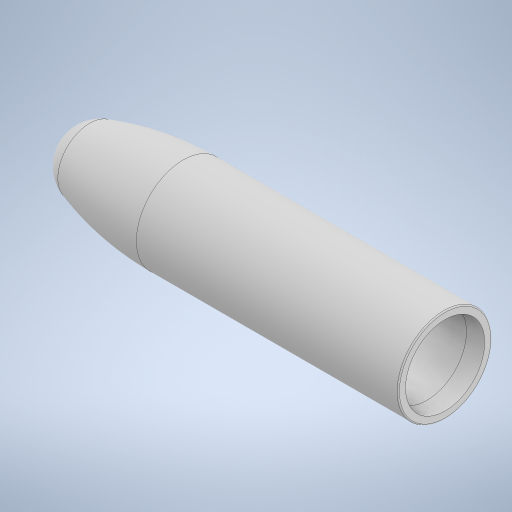
# Autodesk Inventor part: Cap
Saved by Autodesk Inventor 2024 (Build 280153000, 153)
## iProperties
Created: 2024-10-19
Part Number: Cap
Material: Generic
Document SubType Name: Modeling
Designer: Emil
Density: 1 g/cm^3
Appearance: Default
Author: Emil
Autodesk Inventor part; units mm, degrees
ref_plane "YZ Plane" through (0, 0, 0) normal (1, 0, 0) x (0, 1, 0)
ref_plane "XZ Plane" through (0, 0, 0) normal (0, 1, 0) x (-1, 0, 0)
ref_plane "XY Plane" through (0, 0, 0) normal (0, 0, 1) x (1, 0, 0)
sketch "Sketch1" plane through (0, 0, 0) normal (0, 0, 1) x (1, 0, 0)
  line L0 (-32.3906, 7.996) -> (-32.3906, -0.004) construction
  line L1 (-40.3906, -0.004) -> (-32.3906, -0.004) construction
  line L2 (61.6987, -0.004) -> (-73.3826, -0.004) construction
  line L3 (24.6094, 8.046) -> (24.6094, 6.796)
  line L4 (-40.3906, -0.004) -> (-39.1406, -0.004)
  line L5 (21.2094, 9.588) -> (21.2094, 3.996) construction
  line L6 (24.6094, 6.796) -> (21.4757, 6.7961)
  line L7 (24.6094, 8.046) -> (-20.3906, 8.046)
  line L8 (-40.3906, -0.004) -> (-40.3906, 3.996)
  arc A0 (-20.3906, 8.046) -> (-40.3906, 3.996) centre (-20.3906, -43.3617) ccw
  line L9 (20.9432, 6.7961) -> (-22.0568, 6.7961)
  line L10 (-39.1406, -0.004) -> (-39.1406, 2.996)
  arc A1 (-22.0568, 6.7961) -> (-39.1406, 2.996) centre (-20.84, -38.9748) ccw
  line L11 (20.9432, 6.7961) -> (21.4757, 6.7961)
  point P0 (0, 0)
  point P1 (-32.3906, 6.746)
  dimension "d3" = 1.25
  dimension "d4" = 65
  dimension "d6" = 6.8
  dimension "d7" = 8.05
  dimension "d8" = 3.4
  dimension "d12" = 45
  dimension "d13" = 4
  dimension "d14" = 3
  dimension "d16" = 43
  constraints: 24 end point, 5 horizontal, 4 point on circle, 4 vertical, 3 point on line, 2 centre point, 1 collinear, 1 horizontal alignment, 1 tangent
  measures "d3" distance of L3.start L3.end
  measures "d4" horizontal distance of L3.start L1.start
  measures "d6" distance from line of L2 L3.end
  measures "d7" distance from line of L2 L3.start
  measures "d8" distance between parallel lines of L3 L5
  measures "d12" distance of L3.start L7.end
  measures "d13" distance of L1.start L8.end
  measures "d14" distance of L4.end L10.end
  measures "d16" distance of L9.start L9.end
revolve "Revolution1" add sketch "Sketch1" angle 360 about axis through (61.6987, -0.004, 0) along (-1, 0, 0)
fillet "Fillet1" radius 0.2 1 edges at (24.6094, -8.054, 0)
fillet "Fillet2" radius 5.7 1 edges at (-40.3906, -4.004, 0)
fillet "Fillet3" radius 3.9 1 edges at (-39.1406, -3.004, 0)
body "Solid1"
